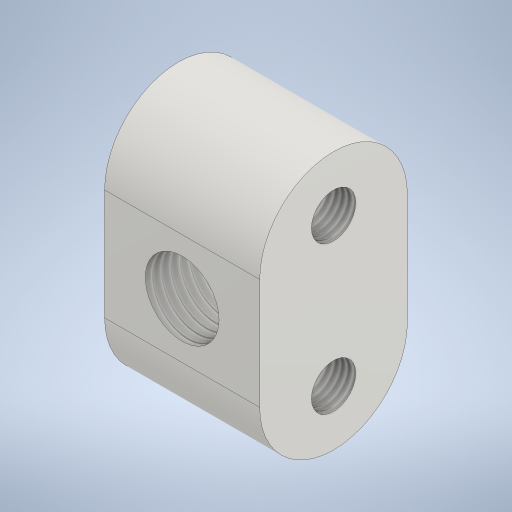
# Autodesk Inventor part: Junção Fuso
Saved by Autodesk Inventor 2024 (Build 280153000, 153)
## iProperties
Created: 2024-06-01
Part Number: Junção Fuso
Material: Steel AISI 1050
Document SubType Name: Modeling
Designer: Pedro
Density: 7.85 g/cm^3
Appearance: Steel
Mass: 988.967 g
Surface Area: 224.566 cm^2
Volume: 125.983 cm^3
Author: Pedro
Autodesk Inventor part; units mm, degrees
ref_plane "YZ Plane" through (0, 0, 0) normal (1, 0, 0) x (0, 1, 0)
ref_plane "XZ Plane" through (0, 0, 0) normal (0, 1, 0) x (-1, 0, 0)
ref_plane "XY Plane" through (0, 0, 0) normal (0, 0, 1) x (1, 0, 0)
sketch "Sketch2" plane through (0, 0, 0) normal (1, 0, 0) x (0, 1, 0)
  line L0 (35, 20) -> (35, -20)
  line L1 (35, -20) -> (-35, -20)
  line L2 (-35, -20) -> (-35, 20)
  line L3 (-35, 20) -> (35, 20)
  point P0 (0, 0)
  dimension "d11" = 40
  dimension "d12" = 70
  dimension "d13" = 35
  dimension "d14" = 20
  constraints: 8 end point, 2 parallel, 1 perpendicular, 1 vertical
  measures "d11" distance of L0.start L0.end
  measures "d12" distance of L0.end L1.end
  measures "d13" distance from line of point (0, 0) L0
  measures "d14" vertical distance of point (0, 0) L1.end
extrude "Extrusion2" add sketch "Sketch2" along normal blind 42
full round fillet "Full Round Fillet1" first side at (14, 11.6667, 20) centre faces at (14, 35, -6.6667) second side at (14, -11.6667, -20)
full round fillet "Full Round Fillet2" first side at (28, -1.6666, 20) centre faces at (14, -35, 6.6667) second side at (28, -18.3333, -20)
sketch "Sketch3" plane through (42, 15, -20) normal (0, 0, -1) x (-1, 0, 0)
  circle A0 centre (21, -15) radius 10
  line L0 (42, -30) -> (42, 0) projected
  point P0 (42, -15)
  point P1 (42, -15)
  dimension "d15" = 20
  dimension "d16" = 21
  constraints: 1 centre point, 1 midpoint
  measures "d15" diameter of A0
  measures "d16" distance of point (42, -15) A0.centre
sketch "Sketch4" plane through (42, 0, 0) normal (1, 0, 0) x (0, 0, -1)
  circle A0 centre (0, -20) radius 6
  circle A1 centre (0, 20) radius 6
  point P0 (0, 0)
  dimension "d17" = 12
  dimension "d18" = 12
  dimension "d31" = 40
  dimension "d32" = 20
  constraints: 2 centre point
  measures "d17" diameter of A0
  measures "d18" diameter of A1
  measures "d31" distance of A0.centre A1.centre
  measures "d32" distance of point (0, 0) A0.centre
extrude "Extrusion3" cut sketch "Sketch3" against normal blind 42
extrude "Extrusion4" cut sketch "Sketch4" against normal blind 42
thread "Thread1" size "M12x1.75" class "6H" standard "ANSI Metric M Profile" full length
thread "Thread2" size "M12x1.75" class "6H" standard "ANSI Metric M Profile" full length
thread "Thread4" size "M20x2.5" class "6H" standard "ANSI Metric M Profile" full length
body "Solid2"
